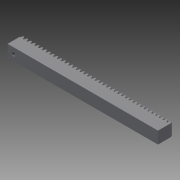
# Autodesk Inventor part: RGEAL1.0HT-125-A5
Saved by Autodesk Inventor 2014 SP2 (Build 180246200, 246)
## iProperties
Created: 2019-03-13
Part Number: RGEAL1.0HT-125-A5
Material: Generic
Catalog Web Link: www.cadenas.de
Description: RGEAL, RGEABL, RGEASL, RGEAML-Rack Gears L Dimension Configurable (One End Machined) - Pressure Angle 20 - Hole Position Configurable
Vendor: MISUMI
Document SubType Name: Modeling
Designer: psadmin
Manufacturer: MISUMI
Mass: 13.6655 g
Surface Area: 66.8284 cm^2
Volume: 13.6655 cm^3
Density: 1 g/cm^3
Appearance: PSOLRGB-175-175-175
Category: PARTsolutions
Company: MISUMI
Title: RGEAL1.0HT-125-A5
Author: Cadenas PARTsolutions
Comments: Rack Gears L Dimension Configurable (One End Machined) - Pressure Angle 20 - Hole Position Configurable
PSOL_IDENT_0: {$CADENAS_DATA\23d-libs\misumi\metric\54_spur_gears\rgeasl.prj},234 {VTYP=3D},{NB=RGEAL1.0HT-125-A5}
PSOL_IDENT_1: ,{LINA=RGEAL1.0HT-125-A5},{NN=RGEAL, RGEABL, RGEASL, RGEAML},{DATE=30.03.2018 07:33:13},{GEOMDATE=05
PSOL_IDENT_2: .09.2016 07:15:33},{VERSION=},{LINEID=30},{WBVAR=MAT,HM,L,A,B,C,ALT1,ALT2,MS},{WBNUMERIC=L,A,B,C,MS}
PSOL_IDENT_3: {NB=RGEAL1.0HT-125-A5},{LINA=RGEAL1.0HT-125-A5},{KT=DUMMY},{PN=RGEAL1.0HT-125-A5},{MAT=2},{MATALG='
PSOL_IDENT_4: 2', '1045 Carbon Steel Equivalent','3', '304 Stainless Steel', '4', 'MC Nylon'},{TYPE=RGEAL},{MOD=1.
PSOL_IDENT_5: 0},{MOD1=1.0},{HM=HT},{HMALG='N', 'No Hole Machining', 'HT', 'Back Tapped', 'ST', 'Side Tapped', 'Z'
PSOL_IDENT_6: , 'Side Counterbore'},{L=125},{LALG=[20:480/1]},{DD21=6.5},{M12=3},{M1=3},{A=5},{AALG=[5:120/1]},{AM
PSOL_IDENT_7: IN=5},{AMAX=120},{B=0},{BALG=0,[5:115/1]},{BMIN=5},{BMAX=115},{C=0},{CALG=0},{CMIN=5},{CMAX=115},{PI
PSOL_IDENT_8: TCH=3.1416},{W=10},{H=12},{HH=11.0},{DD1=3.5},{DD2=6.5},{Z1=3.5},{M=M3},{ALT1= },{ALT1ALG= ' ', 'N/A'
PSOL_IDENT_9: },{ALT2= },{ALT2ALG= ' ', 'N/A' },{ALT2ALGMAX=120},{MS=0},{MSALG=00000},{APN=-A5},{BPN=},{CPN=},{MC
PSOL_IDENT_10: PN=},{WMCPN=},{MSPN=},{TED=2.250},{SP=1.5708},{PFP=0.38},{HAP=1},{HFP=1.25},{DEG1=20},{NN=40},{L3=1.
PSOL_IDENT_11: 14937},{NN1=40}
NN: RGEAL, RGEABL, RGEASL, RGEAML
NT: Rack Gears L Dimension Configurable (One End Machined) - Pressure Angle 20 - Hole Position Configurable
NB: RGEAL1.0HT-125-A5
NBSYN: $PN.
LINA: RGEAL1.0HT-125-A5
PN: RGEAL1.0HT-125-A5
MAT: 1045 Carbon Steel Equivalent
MOD: 1.0
HM: Back Tapped
L: 125
A: 5
B: 0
C: 0
PITCH: 3.1416
W: 10
H: 12
HH: 11
DD1: 3.5
DD2: 6.5
Z1: 3.5
M: M3
ALT1: N/A
ALT2: N/A
MS: 0
SUPPLIER: MISUMI
ARTICLENO: RGEAL1.0HT-125-A5
BOMINFO: RGEAL1.0HT-125-A5
CREATOR: CADENAS GmbH
Autodesk Inventor part; units mm, degrees
ref_plane "YZ Plane" through (0, 0, 0) normal (1, 0, 0) x (0, 1, 0)
ref_plane "XZ Plane" through (0, 0, 0) normal (0, 1, 0) x (-1, 0, 0)
ref_plane "XY Plane" through (0, 0, 0) normal (0, 0, 1) x (1, 0, 0)
sketch "Sketch_1" plane through (0, 0, 0) normal (0, 0, 1) x (1, 0, 0)
  line L0 (0, 12) -> (0, 0)
  line L1 (0, 0) -> (125, 0)
  line L2 (125, 0) -> (125, 12)
  line L3 (125, 12) -> (0, 12)
  constraints: 8 end point
extrude "Extrusion1" add sketch "Sketch_1" along normal blind 10
sketch "Sketch2" plane through (0, 0, 0) normal (0, -1, 0) x (1, 0, 0)
  point P0 (5, 5)
hole "Hole1" at (5, 0, 5) direction (0, 1, 0) diameter 2.459 depth 5.1401 tip angle 120 countersink diameter 3 countersink angle 90 thread size "M3x0.5" class "6H" standard "ISO Metric profile"
sketch "Sketch_4" plane through (0, 0, 5) normal (0, 0, 1) x (1, 0, 0)
  line L0 (5, 0) -> (5, 6.05)
  line L1 (5, 6.05) -> (6.2295, 5.1891)
  line L2 (6.2295, 5.1891) -> (6.2295, 0.2705)
  line L3 (6.2295, 0.2705) -> (6.5, 0)
  line L4 (6.5, 0) -> (5, 0)
  line L5 (5, 0) -> (5, 6.05)
  constraints: 12 end point
revolve "Revolution1" cut sketch "Sketch_4" angle 360 about axis through (5, 0, 5) along (0, -1, 0)
thread "Thread1" size "M3x0.5" class "6H" standard "ISO Metric profile" length 4.2295
sketch "Sketch_21" plane through (0, 0, 0) normal (0, 0, 1) x (1, 0, 0)
  line L0 (-1.1494, 12) -> (-0.4214, 10)
  arc A0 (-0.4214, 10) -> (-0.0644, 9.75) centre (-0.0644, 10.13) ccw
  line L1 (-0.0644, 9.75) -> (0.0644, 9.75)
  arc A1 (0.0644, 9.75) -> (0.4214, 10) centre (0.0644, 10.13) ccw
  line L2 (0.4214, 10) -> (1.1494, 12)
  line L3 (1.1494, 12) -> (-1.1494, 12)
  constraints: 8 end point, 4 point on circle, 2 centre point
extrude "Extrusion2" cut sketch "Sketch_21" along normal blind 10
pattern_linear "Rectangular Pattern1" count 41 spacing 3.1416 along (1, 0, 0) of "Extrusion2"
body "Solid1"
